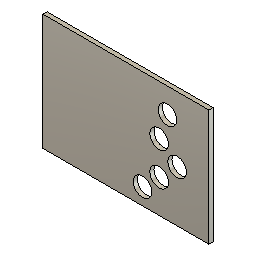
Shooter+Supoert+Plate (Autodesk Fusion 360 design; units mm, degrees)
Autodesk Fusion 360 part; units mm, degrees
sketch "Sketch1" plane through (0, 0, 0) normal (0, 0, 1) x (1, 0, 0)
  line L0 (0, 0) -> (254, 0)
  line L1 (254, 0) -> (254, 177.8)
  line L2 (254, 177.8) -> (0, 177.8)
  line L3 (0, 177.8) -> (0, 0)
  circle A0 centre (177.8, 50.8) radius 14.2748
  circle A1 centre (205.2911, 77.9517) radius 14.2748
  circle A2 centre (177.8, 101.6) radius 14.2748
  circle A3 centre (152.4, 25.4) radius 14.2748
  circle A4 centre (190.5, 139.7) radius 14.2748
  dimension "d1" = 254
  dimension "d2" = 177.8
  dimension "d3" = 28.5496
  dimension "d4" = 177.8
  dimension "d5" = 50.8
  dimension "d6" = 28.5496
  dimension "d7" = 28.5496
  dimension "d8" = 28.5496
  dimension "d9" = 28.5496
  constraint horizontal L0
  constraint vertical L1
  constraint horizontal L2
  constraint vertical L3
  constraint coincident L0.start L3.end
  measures "d1" distance of L0.start L0.end
  measures "d2" distance of L0.start L2.end
  measures "d3" diameter of A0
  measures "d4" distance of L3 A0.centre
  measures "d5" distance of L0 A0.centre
  measures "d6" diameter of A1
  measures "d7" diameter of A2
  measures "d8" diameter of A3
  measures "d9" diameter of A4
extrude "Extrude1" add sketch "Sketch1" along normal blind 6.35
